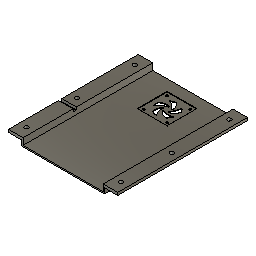
1-CBA bottom Cover V3 - part 2of3 v1 (Autodesk Fusion 360 design; units mm, degrees)
Autodesk Fusion 360 part; units mm, degrees
sketch "extrusion" plane through (0, 0, 0) normal (0, 1, 0) x (1, 0, 0)
  line L0 (-82.5, -8) -> (-62.5, -8)
  line L1 (-62.5, -8) -> (-62.5, 0)
  line L2 (-62.5, 0) -> (62.5, 0)
  line L3 (62.5, 0) -> (62.5, -8)
  line L4 (62.5, -8) -> (82.5, -8)
  line L5 (-60.5, -12) -> (-60.5, -2)
  line L6 (-60.5, -2) -> (60.5, -2)
  line L7 (60.5, -2) -> (60.5, -12)
  line L8 (-82.5, -12) -> (-60.5, -12)
  line L9 (60.5, -12) -> (82.5, -12)
  line L10 (-82.5, -8) -> (-82.5, -12)
  line L11 (82.5, -8) -> (82.5, -12)
  dimension "d1" = 125
  dimension "d2" = 8
  dimension "d3" = 20
  dimension "d4" = 8
  dimension "d5" = 20
  measures "d2" distance of origin
  measures "d4" distance of origin
extrude "Extrude1" add sketch "extrusion" along normal mid plane 196
sketch "top holes" plane through (0, 0, 12) normal (0, 0, 1) x (-1, 0, 0)
  circle A0 centre (71.5, -81.75) radius 3
  line L0 (82.5, -98) -> (60.5, -98)
  dimension "d11" = 6
  dimension "d12" = 16.25
  measures "d11" diameter of A0
extrude "Extrude2" cut sketch "top holes" against normal blind 4
mirror "Mirror1" about plane through (0, 0, 0) normal (1, 0, 0) of "Extrude2"
mirror "Mirror2" about plane through (0, 0, 0) normal (0, 1, 0) of "Extrude2", "Mirror1"
sketch "square undent" plane through (0, 0, 2) normal (0, 0, 1) x (-1, 0, 0)
  line L0 (22.5, -81.5) -> (-22.5, -81.5)
  line L1 (-22.5, -81.5) -> (-22.5, -36.5)
  line L2 (-22.5, -36.5) -> (22.5, -36.5)
  line L3 (22.5, -36.5) -> (22.5, -81.5)
  line L4 (60.5, -98) -> (-60.5, -98)
  dimension "d17" = 45
  dimension "d18" = 45
  dimension "d19" = 16.5
extrude "Extrude3" cut sketch "square undent" against normal blind 1
sketch "square holes" plane through (0, 0, 1) normal (0, 0, 1) x (-1, 0, 0)
  circle A0 centre (17.65, -76.5) radius 1.75
  line L0 (22.5, -81.5) -> (-22.5, -81.5)
  line L1 (22.5, -36.5) -> (22.5, -81.5)
  line L2 (-22.5, -36.5) -> (22.5, -81.5) construction
  circle A1 centre (0, -59) radius 16
  arc A2 (4.2359, -58.0006) -> (0, -43) centre (-16.1329, -55.654) ccw
  arc A3 (6.0614, -58.6697) -> (7.9315, -45.1043) centre (-7.0111, -49.9559) ccw
  arc A4 (4.2359, -58.0006) -> (6.0614, -58.6697) centre (5.2293, -58.115) ccw
  dimension "d22" = 3.5
  dimension "d23" = 5
  dimension "d24" = 4.85
  dimension "d25" = 32
  dimension "d26" = 1
  dimension "d35" = 5.2293
  dimension "d36" = 7.9315
  dimension "d37" = 15.7105
  dimension "d38" = 20.5035
  dimension "d39" = 0.885
  measures "d22" diameter of A0
  measures "d25" diameter of A1
  measures "d26" radius of A4
  measures "d35" distance of origin
  measures "d36" distance of origin
  measures "d37" radius of A3
  measures "d38" radius of A2
  measures "d39" distance of origin
extrude "Extrude4" cut sketch "square holes" against normal blind 1 contours A0
ref_plane "WorkPlane1" through (0, 59, 1.5) normal (0, -1, 0) x (-1, 0, 0)
mirror "Mirror3" about plane through (0, 59, 1.5) normal (0, -1, 0) of "Extrude4"
mirror "Mirror4" about plane through (0, 0, 0) normal (1, 0, 0) of "Extrude4", "Mirror3"
extrude "Extrude5" cut sketch "square holes" against normal blind 1 contours A1 A2 A3 A4 picked at (5.7365, -46.2771)
pattern_circular "C-Pattern1" count 5 over 360 about axis through (0, 59, 1) along (0, 0, -1) of "Extrude5"
sketch "midhole" plane through (0, 0, 12) normal (0, 0, 1) x (-1, 0, 0)
  circle A0 centre (71.5, 5.25) radius 3
  circle A1 centre (71.5, -81.75) radius 3
  dimension "d40" = 81
extrude "Extrude6" cut sketch "midhole" against normal blind 4 contours A0
mirror "Mirror5" about plane through (0, 0, 0) normal (1, 0, 0) of "Extrude6"
sketch "Sketch6" plane through (0, 0, 12) normal (0, 0, 1) x (-1, 0, 0)
  line L0 (60.5, 22.5) -> (82.5, 22.5)
  line L1 (82.5, 22.5) -> (82.5, 17.5)
  line L2 (82.5, 17.5) -> (60.5, 17.5)
  line L3 (60.5, 17.5) -> (60.5, 22.5)
  line L4 (60.5, 98) -> (60.5, -98)
  line L5 (82.5, 98) -> (82.5, -98)
  line L6 (60.5, 98) -> (82.5, 98)
  dimension "d44" = 5
  dimension "d45" = 75.5
  measures "d44" distance of origin
  measures "d45" distance of L0 L6
extrude "Extrude7" cut sketch "Sketch6" against normal blind 4 contours L0 L1 L2 L3 L4 L5
